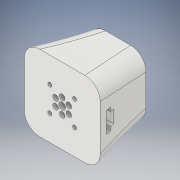
# Autodesk Inventor part: AA034
Saved by Autodesk Inventor 2017 SP1 (Build 210196100, 196)
## iProperties
Created: 2017-09-29
Part Number: AA034
Material: ABS Plastic
Document SubType Name: Modeling
Designer: Zach
Density: 1.06 g/cm^3
Appearance: CR White
Author: Zach
Autodesk Inventor part; units mm, degrees
ref_plane "XZ Plane" through (0, 0, 0) normal (0, 1, 0) x (-1, 0, 0)
ref_plane "XY Plane" through (0, 0, 0) normal (0, 0, 1) x (1, 0, 0)
sketch "Sketch1" plane through (0, 0, 0) normal (0, 0, 1) x (1, 0, 0)
  line L0 (0, 0) -> (70, 0)
  line L1 (70, 0) -> (70, 77.5)
  line L2 (70, 77.5) -> (0, 77.5)
  line L3 (0, 77.5) -> (0, 0)
  dimension "d0" = 70
  dimension "d1" = 77.5
  constraints: 8 end point, 2 parallel, 1 horizontal, 1 perpendicular
  measures "d0" distance of L2.end L1.end
  measures "d1" distance of L1.end L0.end
extrude "Extrusion1" add sketch "Sketch1" along normal blind 70
sketch "Sketch3" plane through (0, 0, 70) normal (0, 0, 1) x (1, 0, 0)
  line L0 (0, 0) -> (70, 0) projected
  line L1 (70, 77.5) -> (0, 77.5) projected
  line L2 (70, 0) -> (35, 0)
  line L3 (35, 0) -> (35, 77.5)
  line L4 (35, 77.5) -> (70, 77.5)
  line L5 (70, 77.5) -> (70, 0)
  constraints: 8 end point, 2 parallel, 1 horizontal, 1 midpoint, 1 perpendicular
extrude "Extrusion3" cut sketch "Sketch3" against normal through all
sketch "Sketch4" plane through (0, 77.5, 70) normal (0, 1, 0) x (1, 0, 0)
  line L0 (0, 70) -> (0, 0) projected
  line L1 (0, 0) -> (-12.5, 0)
  line L2 (35, 70) -> (0, 70) projected
  arc A0 (-12.5, 0) -> (0, 70) centre (-1137.8005, 237.0626) ccw
  line L3 (-12.5, -10) -> (35, -10) construction
  dimension "d9" = 1150
  dimension "d54" = 47.5
  dimension "d55" = 10
  constraints: 4 end point, 2 horizontal, 2 point on circle, 2 vertical alignment, 1 centre point
  measures "d9" radius of A0
  measures "d54" distance of L3.start L3.end
  measures "d55" distance between parallel lines of L1 L3
extrude "Extrusion4" add sketch "Sketch4" against normal blind 77.5
sketch "Sketch5" plane through (35, 0, 70) normal (1, 0, 0) x (0, 0, -1)
  line L0 (0, 77.5) -> (0, 86.25)
  line L1 (0, 0) -> (0, -8.75)
  line L2 (0, 0) -> (0, 77.5) projected
  line L3 (70, 77.5) -> (70, 0) projected
  arc A0 (0, 86.25) -> (70, 77.5) centre (177.5728, 1222.4577) ccw
  arc A1 (70, 0) -> (0, -8.75) centre (177.5728, -1144.9577) ccw
  line L4 (0, 77.5) -> (70, 77.5) projected
  line L5 (70, 0) -> (0, 0) projected
  line L6 (-10, 86.25) -> (-10, -8.75) construction
  point P0 (-10, 38.75)
  point P1 (0, 38.75)
  dimension "d14" = 1150
  dimension "d15" = 1150
  dimension "d52" = 10
  dimension "d53" = 95
  constraints: 6 end point, 4 point on circle, 3 horizontal alignment, 3 vertical, 2 centre point, 2 midpoint
  measures "d14" radius of A0
  measures "d15" radius of A1
  measures "d52" distance between parallel lines of L2 L6
  measures "d53" distance of L6.start L6.end
extrude "Extrusion5" add sketch "Sketch5" against normal blind 55 contours L0 A0 L4 | L5 A1 L1
sketch "Sketch6" plane through (-20, 0, 0) normal (0, 1, 0) x (1, 0, 0)
  line L0 (20, 0) -> (0, 0) projected
  line L1 (0, -70) -> (0, 0) projected
  arc A0 (7.5, -70) -> (20, 0) centre (-1117.8005, 167.0626) ccw projected
  line L2 (7.5, -70) -> (0, -70) projected
extrude "Extrusion6" cut sketch "Sketch6" along normal through all both and the other way through all
fillet "Fillet3" radius 19.35 2 edges at (-5.7463, 81.368, 35.3063) (-5.7463, -3.868, 35.3063)
sketch "Sketch39" plane through (0, 0, 70) normal (0, 0, 1) x (1, 0, 0)
  circle A0 centre (19.5, 54.25) radius 2.5
  circle A1 centre (19.5, 23.25) radius 2.5
  line L0 (35, 86.25) -> (35, -8.75) construction
  line L1 (35, 77.5) -> (35, 0) projected
  circle A2 centre (35, 38.75) radius 4.25
  line L2 (19.5, 54.25) -> (19.5, 23.25) construction
  point P0 (0, 0)
  point P1 (19.5, 38.75)
  dimension "d138" = 5
  dimension "d139" = 5
  dimension "d140" = 8.5
  dimension "d141" = 31
  dimension "d142" = 15.5
  constraints: 3 centre point, 3 midpoint, 2 end point, 1 horizontal alignment, 1 vertical, 1 vertical alignment
  measures "d138" diameter of A0
  measures "d139" diameter of A1
  measures "d140" diameter of A2
  measures "d141" distance of L2.start L2.end
  measures "d142" distance from line of A2.centre L2
extrude "Extrusion33" cut sketch "Sketch39" against normal through all
ref_plane "Work Plane7" through (0, 0, 60) normal (0, 0, 1) x (1, 0, 0)
sketch "Sketch41" plane through (0, 0, 60) normal (0, 0, 1) x (1, 0, 0)
  arc A0 (35, 43) -> (35, 34.5) centre (35, 38.75) ccw projected
  circle A1 centre (35, 38.75) radius 13
  point P0 (0, 0)
  dimension "d151" = 26
  constraints: 1 centre point, 1 coincident
  measures "d151" diameter of A1
extrude "Extrusion34" cut sketch "Sketch41" against normal blind 6
sketch "Sketch42" plane through (0, 0, 60) normal (0, 0, -1) x (-1, 0, 0)
  arc A0 (-35, 34.5) -> (-35, 43) centre (-35, 38.75) ccw projected
  circle A1 centre (-35, 38.75) radius 8
  point P0 (0, 0)
  dimension "d154" = 16
  constraints: 1 centre point, 1 coincident
  measures "d154" diameter of A1
extrude "Extrusion35" cut sketch "Sketch42" along normal blind 11
mirror "Mirror1" about plane through (35, 0, 70) normal (1, 0, 0)
ref_plane "Work Plane8" through (35, 86.25, 70) normal (1, 0, 0) x (0, 1, 0)
sketch "Sketch43" plane through (35, 86.25, 70) normal (1, 0, 0) x (0, 1, 0)
  line L0 (-34.5, -16) -> (-60.5, -16) projected
  line L1 (-60.5, -10) -> (-34.5, -10) projected
  line L2 (-39.5, -21) -> (-55.5, -21) projected
  line L3 (-55.5, -16) -> (-39.5, -16) projected
  line L4 (-55.5, -16) -> (-55.5, -21) projected
  line L5 (-60.5, -10) -> (-60.5, -16) projected
  line L6 (-39.5, -16) -> (-39.5, -21) projected
  line L7 (-34.5, -10) -> (-34.5, -16) projected
  point P0 (-86.25, -70)
extrude "Extrusion36" cut sketch "Sketch43" along normal through all
sketch "Sketch44" plane through (0, 0, 60) normal (0, 0, -1) x (-1, 0, 0)
  circle A0 centre (-35, 38.75) radius 4.25 projected
  circle A1 centre (-35, 48.2797) radius 1.5
  circle A2 centre (-43.253, 43.5149) radius 1.5
  circle A3 centre (-43.253, 33.9851) radius 1.5
  circle A4 centre (-35, 29.2203) radius 1.5
  circle A5 centre (-26.747, 33.9851) radius 1.5
  circle A6 centre (-26.747, 43.5149) radius 1.5
  point P0 (0, 0)
  dimension "d159" = 3
  dimension "d160" = 9.5297
  dimension "d163" = 360
  constraints: 6 centre point, 1 vertical alignment, 13 other
  measures "d159" diameter of A1
  measures "d160" distance of A0.centre A1.centre
extrude "Extrusion37" cut sketch "Sketch44" against normal through all contours A1 | A2 | A3 | A4 | A5 | A6
sketch "Sketch45" plane through (0, 0, 70) normal (0, 0, 1) x (1, 0, 0)
  circle A0 centre (35, 29.2203) radius 1.5 construction
  circle A1 centre (35, 29.2203) radius 3.5
  circle A2 centre (35, 38.75) radius 4.25 projected
  circle A3 centre (43.253, 33.9851) radius 3.5
  circle A4 centre (43.253, 43.5149) radius 3.5
  circle A5 centre (35, 48.2797) radius 3.5
  circle A6 centre (26.747, 43.5149) radius 3.5
  circle A7 centre (26.747, 33.9851) radius 3.5
  point P0 (0, 0)
  dimension "d167" = 7
  dimension "d170" = 360
  constraints: 6 centre point, 1 coincident, 13 other
  measures "d167" diameter of A1
extrude "Extrusion38" cut sketch "Sketch45" against normal blind 5
body "Solid1"
